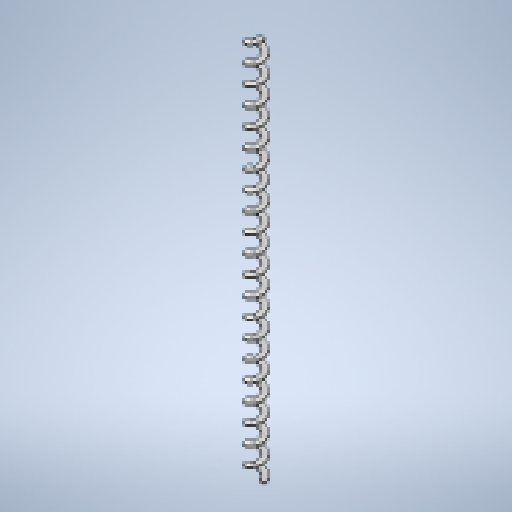
# Autodesk Inventor part: NVPH-401 auger
Saved by Autodesk Inventor 2025.1 (Build 291241020, 241B)
## iProperties
Created: 2024-12-03
Part Number: NVPH-401 auger
Material: Generic
Document SubType Name: Modeling
Designer: user
Density: 1 g/cm^3
Appearance: Default
Author: user
Autodesk Inventor part; units mm, degrees
ref_plane "YZ Plane" through (0, 0, 0) normal (1, 0, 0) x (0, 1, 0)
ref_plane "XZ Plane" through (0, 0, 0) normal (0, 1, 0) x (-1, 0, 0)
ref_plane "XY Plane" through (0, 0, 0) normal (0, 0, 1) x (1, 0, 0)
sketch "Sketch2" plane through (0, 0, 0) normal (0, 1, 0) x (-1, 0, 0)
  line L0 (-15, 4) -> (-45, 4)
  line L1 (-45, 4) -> (-45, -4)
  line L2 (-45, -4) -> (-15, -4)
  line L3 (-15, -4) -> (-15, 4)
  line L4 (-15, 4) -> (-45, -4) construction
  line L5 (-45, 4) -> (-15, -4) construction
  line L6 (0, 0) -> (0, 57.5902)
  point P0 (-30, 0)
  dimension "d1" = 8
  dimension "d11" = 30
  dimension "d12" = 90
  constraints: 14 end point, 2 midpoint, 2 parallel, 1 horizontal, 1 horizontal alignment, 1 perpendicular, 1 vertical
  measures "d1" distance of L1.end L0.end
  measures "d11" diameter of L3 L6
  measures "d12" diameter of L1 L6
coil "Coil1" sketch "Sketch2" operation add axis through (0, 0, -10) along (0, 0, 1) pitch 90 turns 21 hand right
body "Solid1"
